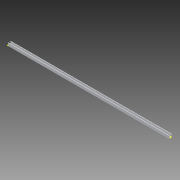
# Autodesk Inventor part: 26in mini C-Channel (rail)
Saved by Autodesk Inventor 2013 (Build 170138000, 138)
## iProperties
Created: 2013-01-27
Part Number: 26in mini C-Channel (rail)
Material: Aluminum 6061
Document SubType Name: Modeling
Designer: Naphat
Density: 2.71 g/cm^3
Mass: 61.8868 g
Surface Area: 322.617 cm^2
Volume: 22.8365 cm^3
Author: Naphat
Autodesk Inventor part; units mm, degrees
ref_plane "YZ Plane" through (0, 0, 0) normal (1, 0, 0) x (0, 1, 0)
ref_plane "XZ Plane" through (0, 0, 0) normal (0, 1, 0) x (-1, 0, 0)
ref_plane "XY Plane" through (0, 0, 0) normal (0, 0, 1) x (1, 0, 0)
sketch "Sketch1" plane through (0, 0, 0) normal (1, 0, 0) x (0, 1, 0)
  line L0 (0, 0) -> (0, -10)
  line L1 (0, -10) -> (10, -10)
  line L2 (10, -10) -> (10, -8.5)
  line L3 (0, 0) -> (10, 0)
  line L4 (10, 0) -> (10, -1.5)
  line L5 (0, -5) -> (1.5, -5) construction
  line L6 (10, -1.5) -> (1.5, -1.5)
  line L7 (1.5, -1.5) -> (1.5, -8.5)
  line L8 (1.5, -8.5) -> (10, -8.5)
  dimension "d0" = 10
  dimension "d1" = 10
  dimension "d2" = 1.5
  dimension "d3" = 10
  dimension "d4" = 1.5
  dimension "d5" = 1.5
  constraints: 18 end point, 5 perpendicular, 3 parallel, 1 midpoint, 1 vertical
  measures "d0" distance of L0.start L0.end
  measures "d1" distance of L0.end L1.end
  measures "d2" distance of L1.end L2.end
  measures "d3" distance of L0.start L3.end
  measures "d4" distance of L3.end L4.end
  measures "d5" distance of L5.start L5.end
extrude "Extrusion1" add sketch "Sketch1" along normal blind 564.7944
sketch "Sketch2" plane through (0, 1.5, -1.5) normal (0, 1, 0) x (1, 0, 0)
  line L0 (0, 7) -> (0, 0) projected
  line L1 (564.7944, 7) -> (564.7944, 0) projected
  line L2 (0, 7) -> (564.7944, 7) projected
  circle A0 centre (550.7944, 3.5) radius 2 projected
  circle A1 centre (550.7944, 136.95) radius 2 projected
  circle A2 centre (550.7944, 3.5) radius 2
  circle A3 centre (14, 3.5) radius 2
  line L3 (0, 0) -> (564.7944, 0) projected
  point P0 (0, -1.5)
  dimension "d8" = 4
  dimension "d9" = 14
  dimension "d10" = 7
  dimension "d11" = 3.5
  dimension "d12" = 4
  dimension "d13" = 14
  constraints: 2 centre point, 1 horizontal alignment
  measures "d8" diameter of A2
  measures "d9" distance from line of A2.centre L1
  measures "d10" distance of L1.start L1.end
  measures "d11" distance from line of L2 A2.centre
  measures "d12" diameter of A3
  measures "d13" distance from line of L0 A3.centre
hole "Hole1" at (550.7944, 1.5, -5) at (14, 1.5, -5) direction (0, -1, 0) diameter 4 end through all
equation "\"d11\" = 0.5 * d10"
equation "\"d13\" = d9"
body "Solid1"
